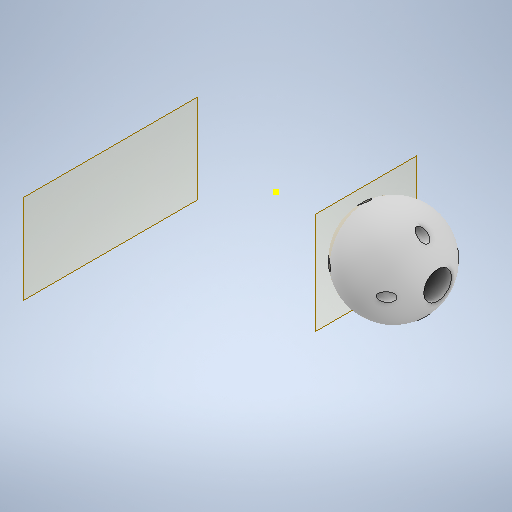
# Autodesk Inventor part: Part3
Saved by Autodesk Inventor 2025.2 (Build 292293000, 293)
## iProperties
Created: 2025-04-03
Part Number: Part3
Material: Generic
Document SubType Name: Modeling
Designer: avnr2
Density: 1 g/cm^3
Appearance: Default
Author: avnr2
Autodesk Inventor part; units mm, degrees
ref_plane "XZ Plane" through (0, 0, 0) normal (0, 1, 0) x (-1, 0, 0)
ref_plane "XY Plane" through (0, 0, 0) normal (0, 0, 1) x (1, 0, 0)
sketch "Sketch1" plane through (0, 0, 0) normal (1, 0, 0) x (0, 1, 0)
  point P0 (0, 0)
sketch "Sketch2" plane through (0, 0, 0) normal (0, 1, 0) x (-1, 0, 0)
  point P0 (0, 0)
sketch "Sketch3" plane through (0, 0, 0) normal (0, 1, 0) x (-1, 0, 0)
  arc A0 (-5, 0) -> (5, 0) centre (0, 0) ccw
  line L0 (5, 0) -> (-5, 0)
  dimension "d0" = 10
  constraints: 2 end point, 2 point on circle, 1 centre point, 1 coincident, 1 horizontal
  measures "d0" diameter of A0
revolve "Revolution1" add sketch "Sketch3" angle 360 about axis through (-5, 0, 0) along (1, 0, 0)
ref_plane "Work Plane1" through (-12.7, 0, 0) normal (1, 0, 0) x (0, 1, 0)
sketch "Sketch4" plane through (-12.7, 0, 0) normal (1, 0, 0) x (0, 1, 0)
  point P0 (0, 0)
sketch "Sketch5" plane through (-12.7, 0, 0) normal (1, 0, 0) x (0, 1, 0)
  point P0 (0, 0)
sketch "Sketch6" plane through (-12.7, 0, 0) normal (1, 0, 0) x (0, 1, 0)
  circle A0 centre (0, 0) radius 1.5
  circle A1 centre (0, 0) radius 3.8495 construction
  circle A2 centre (0, 3.8495) radius 0.5
  circle A3 centre (0, 0) radius 3.8495 construction
  circle A4 centre (-3.8495, 0) radius 0.5
  circle A5 centre (0, 0) radius 3.8495 construction
  circle A6 centre (0, -3.8495) radius 0.5
  circle A7 centre (0, 0) radius 3.8495 construction
  circle A8 centre (3.8495, 0) radius 0.5
  dimension "d3" = 3
  dimension "d4" = 1
  dimension "d7" = 360
  constraints: 5 centre point, 4 coincident, 2 horizontal alignment, 2 vertical alignment, 27 other
  measures "d3" diameter of A0
  measures "d4" diameter of A2
extrude "Extrusion1" cut sketch "Sketch6" along normal blind 100
sketch "Sketch7" plane through (0, 0, 0) normal (0, 0, 1) x (1, 0, 0)
  point P0 (0, 0)
ref_plane "Work Plane2" through (-3, 0, 0) normal (1, 0, 0) x (0, 1, 0)
sketch "Sketch8" plane through (-3, 0, 0) normal (1, 0, 0) x (0, 1, 0)
  point P0 (0, 0)
body "Solid1"
